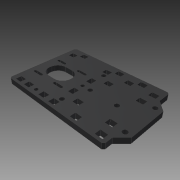
# Autodesk Inventor part: x_motor_back
Saved by Autodesk Inventor 2014 (Build 180170000, 170)
## iProperties
Created: 2013-11-30
Part Number: x_motor_back
Material: Generic
Document SubType Name: Modeling
Designer: buben
Density: 1 g/cm^3
Appearance: Anodized - Dark Gray
Author: buben
Subject: Laser Cutted
Autodesk Inventor part; units mm, degrees
ref_plane "YZ Plane" through (0, 0, 0) normal (1, 0, 0) x (0, 1, 0)
ref_plane "XZ Plane" through (0, 0, 0) normal (0, 1, 0) x (-1, 0, 0)
ref_plane "XY Plane" through (0, 0, 0) normal (0, 0, 1) x (1, 0, 0)
sketch "Sketch1" plane through (0, 0, 0) normal (0, 0, 1) x (1, 0, 0)
  line L0 (0, 0) -> (125, 0)
  line L1 (125, 87.5) -> (0, 87.5)
  line L2 (0, 87.5) -> (0, 0)
  line L3 (12.7, 56) -> (43.7, 56) construction
  line L4 (43.7, 56) -> (43.7, 25) construction
  line L5 (43.7, 25) -> (12.7, 25) construction
  line L6 (12.7, 25) -> (12.7, 56) construction
  line L7 (7.7, 56) -> (17.7, 56) construction
  line L8 (7.7, 54.3) -> (17.7, 54.3)
  line L9 (17.7, 57.7) -> (7.7, 57.7)
  arc A0 (7.7, 57.7) -> (7.7, 54.3) centre (7.7, 56) ccw
  arc A1 (17.7, 54.3) -> (17.7, 57.7) centre (17.7, 56) ccw
  line L10 (38.7, 56) -> (48.7, 56) construction
  line L11 (38.7, 54.3) -> (48.7, 54.3)
  line L12 (48.7, 57.7) -> (38.7, 57.7)
  arc A2 (38.7, 57.7) -> (38.7, 54.3) centre (38.7, 56) ccw
  arc A3 (48.7, 54.3) -> (48.7, 57.7) centre (48.7, 56) ccw
  line L13 (7.7, 25) -> (17.7, 25) construction
  line L14 (7.7, 23.3) -> (17.7, 23.3)
  line L15 (17.7, 26.7) -> (7.7, 26.7)
  arc A4 (7.7, 26.7) -> (7.7, 23.3) centre (7.7, 25) ccw
  arc A5 (17.7, 23.3) -> (17.7, 26.7) centre (17.7, 25) ccw
  line L16 (38.7, 25) -> (48.7, 25) construction
  line L17 (38.7, 26.7) -> (48.7, 26.7)
  line L18 (48.7, 23.3) -> (38.7, 23.3)
  arc A6 (38.7, 26.7) -> (38.7, 23.3) centre (38.7, 25) ccw
  arc A7 (48.7, 23.3) -> (48.7, 26.7) centre (48.7, 25) ccw
  line L19 (23.2, 40.5) -> (33.2, 40.5) construction
  line L20 (23.2, 52) -> (33.2, 52)
  line L21 (33.2, 29) -> (23.2, 29)
  arc A8 (23.2, 52) -> (23.2, 29) centre (23.2, 40.5) ccw
  arc A9 (33.2, 29) -> (33.2, 52) centre (33.2, 40.5) ccw
  line L22 (6, 78) -> (14, 78)
  line L23 (14, 78) -> (14, 71.5)
  line L24 (14, 71.5) -> (6, 71.5)
  line L25 (6, 71.5) -> (6, 78)
  line L26 (6, 9.5) -> (14, 9.5)
  line L27 (14, 9.5) -> (14, 3)
  line L28 (14, 3) -> (6, 3)
  line L29 (6, 3) -> (6, 9.5)
  line L30 (125, 71.5) -> (135, 61.5)
  line L31 (135, 61.5) -> (135, 19.5)
  line L32 (135, 19.5) -> (125, 9.5)
  line L33 (125, 0) -> (125, 9.5)
  line L34 (125, 71.5) -> (125, 87.5)
  line L35 (72, 63.5) -> (80, 63.5)
  line L36 (80, 63.5) -> (80, 57)
  line L37 (80, 57) -> (72, 57)
  line L38 (72, 57) -> (72, 63.5)
  line L39 (72, 24) -> (80, 24)
  line L40 (80, 24) -> (80, 17.5)
  line L41 (80, 17.5) -> (72, 17.5)
  line L42 (72, 17.5) -> (72, 24)
  line L43 (0, 67.5) -> (129, 67.5) construction
  line L44 (0, 13.5) -> (129, 13.5) construction
  line L45 (129, 67.5) -> (129, 13.5) construction
  line L46 (17, 84.5) -> (25, 84.5)
  line L47 (25, 84.5) -> (25, 78)
  line L48 (25, 78) -> (17, 78)
  line L49 (17, 78) -> (17, 84.5)
  line L50 (113, 78) -> (121, 78)
  line L51 (121, 78) -> (121, 71.5)
  line L52 (121, 71.5) -> (113, 71.5)
  line L53 (113, 71.5) -> (113, 78)
  line L54 (113, 9.5) -> (121, 9.5)
  line L55 (121, 9.5) -> (121, 3)
  line L56 (121, 3) -> (113, 3)
  line L57 (113, 3) -> (113, 9.5)
  circle A10 centre (128, 60.5) radius 2.75
  circle A11 centre (63, 67.5) radius 2.75
  circle A12 centre (63, 13.5) radius 2.75
  circle A13 centre (128, 20.5) radius 2.75
  line L58 (57, 87.5) -> (57, 0) construction
  line L59 (11.7, 62) -> (54.7, 62) construction
  line L60 (54.7, 62) -> (54.7, 19) construction
  line L61 (54.7, 19) -> (11.7, 19) construction
  line L62 (11.7, 19) -> (11.7, 62) construction
  line L63 (17.7, 25) -> (48.7, 25) construction
  line L64 (110, 63.5) -> (118, 63.5)
  line L65 (118, 63.5) -> (118, 57)
  line L66 (118, 57) -> (110, 57)
  line L67 (110, 57) -> (110, 63.5)
  line L68 (110, 24) -> (118, 24)
  line L69 (118, 24) -> (118, 17.5)
  line L70 (118, 17.5) -> (110, 17.5)
  line L71 (110, 17.5) -> (110, 24)
  line L72 (85, 78) -> (93, 78)
  line L73 (93, 78) -> (93, 71.5)
  line L74 (93, 71.5) -> (85, 71.5)
  line L75 (85, 71.5) -> (85, 78)
  line L76 (85, 9.5) -> (93, 9.5)
  line L77 (93, 9.5) -> (93, 3)
  line L78 (93, 3) -> (85, 3)
  line L79 (85, 3) -> (85, 9.5)
  line L80 (57, 78) -> (65, 78)
  line L81 (65, 78) -> (65, 71.5)
  line L82 (65, 71.5) -> (57, 71.5)
  line L83 (57, 71.5) -> (57, 78)
  line L84 (57, 9.5) -> (65, 9.5)
  line L85 (65, 9.5) -> (65, 3)
  line L86 (65, 3) -> (57, 3)
  line L87 (57, 3) -> (57, 9.5)
  line L88 (68, 84.5) -> (76, 84.5)
  line L89 (76, 84.5) -> (76, 78)
  line L90 (76, 78) -> (68, 78)
  line L91 (68, 78) -> (68, 84.5)
  line L92 (96, 84.5) -> (104, 84.5)
  line L93 (104, 84.5) -> (104, 78)
  line L94 (104, 78) -> (96, 78)
  line L95 (96, 78) -> (96, 84.5)
  circle A14 centre (71, 40.5) radius 5 construction
  circle A15 centre (103, 40.5) radius 5 construction
  circle A16 centre (103, 40.5) radius 2.75
  circle A17 centre (71, 40.5) radius 2.75
  point P0 (28.2, 40.5)
  point P1 (28.2, 56)
  point P2 (12.7, 40.5)
  point P3 (129, 40.5)
  point P4 (11.7, 40.5)
  point P5 (33.2, 25)
  point P6 (33.2, 19)
  dimension "d1" = 31
  dimension "d2" = 31
  dimension "d3" = 3.4
  dimension "d4" = 3.4
  dimension "d5" = 3.4
  dimension "d6" = 3.4
  dimension "d7" = 10
  dimension "d8" = 23
  dimension "d9" = 3
  dimension "d10" = 6.5
  dimension "d11" = 6.5
  dimension "d13" = 45
  dimension "d14" = 10
  dimension "d15" = 8
  dimension "d16" = 6.5
  dimension "d17" = 8
  dimension "d18" = 6.5
  dimension "d19" = 4
  dimension "d21" = 8
  dimension "d22" = 8
  dimension "d23" = 7.7
  dimension "d25" = 8
  dimension "d26" = 6.5
  dimension "d27" = 3
  dimension "d28" = 6
  dimension "d29" = 8
  dimension "d30" = 4
  dimension "d31" = 4
  dimension "d32" = 125
  dimension "d33" = 5.5
  dimension "d34" = 5.5
  dimension "d35" = 5.5
  dimension "d36" = 5.5
  dimension "d37" = 7
  dimension "d38" = 11
  dimension "d39" = 7
  dimension "d40" = 11
  dimension "d41" = 62
  dimension "d42" = 68
  dimension "d43" = 43
  dimension "d44" = 43
  dimension "d45" = 8
  dimension "d47" = 8
  dimension "d48" = 10
  dimension "d49" = 8
  dimension "d50" = 20
  dimension "d51" = 8
  dimension "d52" = 20
  dimension "d53" = 8
  dimension "d54" = 8
  dimension "d55" = 3
  dimension "d56" = 3
  dimension "d57" = 15
  dimension "d58" = 10
  dimension "d59" = 10
  dimension "d60" = 5.5
  dimension "d61" = 5.5
  dimension "d62" = 14
  dimension "d63" = 32
  dimension "d96" = 3
  dimension "d97" = 54
  constraints: 202 end point, 49 parallel, 33 collinear, 23 perpendicular, 20 point on circle, 20 tangent, 18 centre point, 18 horizontal, 11 midpoint, 8 point on line, 7 horizontal alignment, 6 coincident, 4 equal length, 3 vertical alignment
  measures "d1" distance of L3.start L3.end
  measures "d2" distance of L3.end L4.end
  measures "d3" distance between parallel lines of L8 L9
  measures "d4" distance between parallel lines of L11 L12
  measures "d5" distance between parallel lines of L14 L15
  measures "d6" distance between parallel lines of L18 L17
  measures "d7" distance of L7.start L7.end
  measures "d8" distance between parallel lines of L21 L20
  measures "d9" distance between parallel lines of L0 L28
  measures "d10" distance of L28.end L26.start
  measures "d11" distance of L24.end L22.start
  measures "d13" angle of L30 L34
  measures "d14" distance between parallel lines of L34 L31
  measures "d15" distance between parallel lines of L35 L24
  measures "d16" distance of L35.end L36.end
  measures "d17" distance between parallel lines of L41 L26
  measures "d18" distance of L39.end L40.end
  measures "d19" distance between parallel lines of L43 L24
  measures "d21" distance of L22.start L22.end
  measures "d22" distance of L27.end L28.end
  measures "d23" distance from line of L2 L7.start
  measures "d25" distance of L46.start L46.end
  measures "d26" distance of L48.end L46.start
  measures "d27" distance between parallel lines of L23 L49
  measures "d28" distance between parallel lines of L2 L29
  measures "d29" distance between parallel lines of L51 L53
  measures "d30" distance between parallel lines of L34 L51
  measures "d31" distance between parallel lines of L44 L26
  measures "d32" distance of L0.start L0.end
  measures "d33" diameter of A13
  measures "d34" diameter of A10
  measures "d35" diameter of A11
  measures "d36" diameter of A12
  measures "d37" distance from line of L31 A10.centre
  measures "d38" vertical distance of A10.centre L30.start
  measures "d39" distance from line of L31 A13.centre
  measures "d40" vertical distance of L32.end A13.centre
  measures "d41" distance from line of L34 A11.centre
  measures "d42" distance between parallel lines of L33 L58
  measures "d43" distance of L59.start L59.end
  measures "d44" distance of L61.end L59.start
  measures "d45" distance of L36.end L37.end
  measures "d47" distance of L64.start L64.end
  measures "d48" distance from line of A10.centre L65
  measures "d49" distance of L72.start L72.end
  measures "d50" distance between parallel lines of L53 L73
  measures "d51" distance of L80.start L80.end
  measures "d52" distance between parallel lines of L75 L81
  measures "d53" distance of L88.start L88.end
  measures "d54" distance of L92.start L92.end
  measures "d55" distance between parallel lines of L81 L91
  measures "d56" distance between parallel lines of L73 L95
  measures "d57" distance between parallel lines of L58 L38
  measures "d58" diameter of A14
  measures "d59" diameter of A15
  measures "d60" diameter of A17
  measures "d61" diameter of A16
  measures "d62" distance from line of L58 A14.centre
  measures "d63" distance from line of L31 A15.centre
  measures "d96" distance between parallel lines of L46 L1
  measures "d97" distance between parallel lines of L44 L43
extrude "Extrusion4" add sketch "Sketch1" along normal blind 6.5
sketch "Sketch4" plane through (0, 0, 6.5) normal (0, 0, 1) x (1, 0, 0)
  arc A0 (33.2, 29) -> (33.2, 52) centre (33.2, 40.5) ccw projected
  line L0 (14, 9.5) -> (14, 3) projected
  line L1 (6, 9.5) -> (14, 9.5) projected
  line L2 (11.7, 62) -> (54.7, 62) construction
  line L3 (54.7, 62) -> (54.7, 19) construction
  line L4 (54.7, 19) -> (11.7, 19) construction
  line L5 (11.7, 19) -> (11.7, 62) construction
  line L6 (57.7, 56) -> (64.2, 56)
  line L7 (64.2, 56) -> (64.2, 48)
  line L8 (64.2, 48) -> (57.7, 48)
  line L9 (57.7, 48) -> (57.7, 56)
  line L10 (57.7, 33) -> (64.2, 33)
  line L11 (64.2, 33) -> (64.2, 25)
  line L12 (64.2, 25) -> (57.7, 25)
  line L13 (57.7, 25) -> (57.7, 33)
  line L14 (50.5, 9.5) -> (42.5, 9.5)
  line L15 (42.5, 9.5) -> (42.5, 3)
  line L16 (42.5, 3) -> (50.5, 3)
  line L17 (50.5, 3) -> (50.5, 9.5)
  line L18 (27.5, 9.5) -> (19.5, 9.5)
  line L19 (19.5, 9.5) -> (19.5, 3)
  line L20 (19.5, 3) -> (27.5, 3)
  line L21 (27.5, 3) -> (27.5, 9.5)
  line L22 (27.5, 9.5) -> (42.5, 3) construction
  line L23 (27.5, 3) -> (42.5, 9.5) construction
  line L24 (64.2, 33) -> (57.7, 48) construction
  line L25 (64.2, 48) -> (57.7, 33) construction
  circle A1 centre (35, 6.25) radius 2.25
  circle A2 centre (60.95, 40.5) radius 2.25
  point P0 (33.2, 62)
  point P1 (11.7, 40.5)
  dimension "d100" = 43
  dimension "d101" = 6.5
  dimension "d102" = 8
  dimension "d103" = 15
  dimension "d104" = 15
  dimension "d105" = 4.5
  dimension "d106" = 4.5
  dimension "d107" = 3
  dimension "d108" = 21
  constraints: 48 end point, 10 parallel, 7 equal length, 6 perpendicular, 5 horizontal, 4 midpoint, 3 collinear, 2 centre point, 2 horizontal alignment, 1 point on line, 1 vertical alignment
  measures "d100" distance of L3.end L4.end
  measures "d101" distance of L18.end L19.end
  measures "d102" distance of L18.start L18.end
  measures "d103" distance between parallel lines of L15 L21
  measures "d104" distance between parallel lines of L8 L10
  measures "d105" diameter of A2
  measures "d106" diameter of A1
  measures "d107" distance between parallel lines of L3 L9
  measures "d108" distance from line of A1.centre L0
extrude "Extrusion5" cut sketch "Sketch4" against normal blind 6.5
chamfer "Chamfer2" distance 2 angle 45 4 edges at (0, 87.5, 3.25) (0, 0, 3.25) (125, 0, 3.25) (125, 87.5, 3.25)
body "Solid2"
